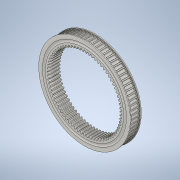
# Autodesk Inventor part: Spur Gear2
Saved by Autodesk Inventor 2020 (Build 240168000, 168)
## iProperties
CustomPartVersion: 1
Created: 2019-05-08
Part Number: Spur Gear2
Material: Steel
Document SubType Name: Modeling
Designer: Connor
Categories: <?xml version="1.0" encoding="UTF-16"?> <MemberInstance><Categories><FamilyTemplate><FamilyTemplateParameter ValueType="xs:double" Id="1" ObjectReferenceKey="da_z" ObjectType="kUserParameterObject"/><FamilyTemplateParameter ValueType="xs:double" Id="2" ObjectReferenceKey="da_b" ObjectType="kUserParameterObject"/><FamilyTemplateParameter ValueType="xs:double" Id="3" ObjectReferenceKey="da_beta" ObjectType="kUserParameterObject"/><FamilyTemplateParameter ValueType="xs:double" Id="4" ObjectReferenceKey="da_da" ObjectType="kUserParameterObject"/><FamilyTemplateParameter ValueType="xs:double" Id="5" ObjectReferenceKey="da_aw" ObjectType="kUserParameterObject"/><FamilyTemplateParameter ValueType="xs:string" Id="6" ObjectReferenceKey="EAIAABAAAAC/AAAAAAAAAIAAAAAAAAAA" ObjectType="83910656" SubObjectId="SurfaceGeometry"/></FamilyTemplate><ParamToTemplateMap><ParamToTemplate CategoryParameter="//CategoryParameter[@InternalName='046C89C9-8512-4d59-83FE-43B91F4F132A']" TemplateParameter="1"/><ParamToTemplate CategoryParameter="//CategoryParameter[@InternalName='2552DF32-E462-4b46-AEBF-C6C7768E72AC']" TemplateParameter="2"/><ParamToTemplate CategoryParameter="//CategoryParameter[@InternalName='C9EE641D-15FC-4fae-A226-E94C4372FDD7']" TemplateParameter="3"/><ParamToTemplate><ParamToTemplate CategoryParameter="//CategoryParameter[@InternalName='00B6519A-459B-49c7-AD84-2E56D39A5744']" ConstantValue="-0.000000"/></ParamToTemplate><ParamToTemplate><ParamToTemplate CategoryParameter="//CategoryParameter[@InternalName='04B31F0E-C7A6-4894-AA32-9629BEFACF47']" ConstantValue="1.000000"/></ParamToTemplate><ParamToTemplate><ParamToTemplate CategoryParameter="//CategoryParameter[@InternalName='43CBEC2E-7847-49e7-A936-2F7889FCB2D9']" ConstantValue="0.250000"/></ParamToTemplate><ParamToTemplate><ParamToTemplate CategoryParameter="//CategoryParameter[@InternalName='B1EFC894-105D-4ebd-86BF-FA20ED196853']" ConstantValue="0.333500"/></ParamToTemplate><ParamToTemplate><ParamToTemplate CategoryParameter="//CategoryParameter[@InternalName='51175063-3D10-4879-93E8-6246FE8B403D']" ConstantValue="2061532430.657340"/></ParamToTemplate><ParamToTemplate><ParamToTemplate CategoryParameter="//CategoryParameter[@InternalName='A3A52E27-4454-46a9-B0BD-C932399B70AF']" ConstantValue="0.300000"/></ParamToTemplate><ParamToTemplate><ParamToTemplate CategoryParameter="//CategoryParameter[@InternalName='91B76062-C214-41d9-B1B9-14D2AB99603D']" ConstantValue="0.127000"/></ParamToTemplate><ParamToTemplate><ParamToTemplate CategoryParameter="//CategoryParameter[@InternalName='374E806E-8B8A-4dda-A9AA-1039D6500AD2']" ConstantValue="7.874016"/></ParamToTemplate><ParamToTemplate><ParamToTemplate CategoryParameter="//CategoryParameter[@InternalName='2D373A89-B862-43d6-8D0B-0CBF12AB9F6C']" ConstantValue="0.253073"/></ParamToTemplate><ParamToTemplate CategoryParameter="//CategoryParameter[@InternalName='37777632-D6A2-4fac-9D53-DB8ACD95C989']" TemplateParameter="4"/><ParamToTemplate CategoryParameter="//CategoryParameter[@InternalName='FD1017F1-B727-4f7e-9707-0F86F1FF9423']" TemplateParameter="5"/><ParamToTemplate><ParamToTemplate CategoryParameter="//CategoryParameter[@InternalName='9E1B4470-B2D3-4ff1-B813-535BB4CDF51A']" ConstantValue="3523220.976809"/></ParamToTemplate><ParamToTemplate><ParamToTemplate CategoryParameter="//CategoryParameter[@InternalName='F8452263-BFF6-458c-9FB1-07C4B99E95CD']" ConstantValue="11397033.805607"/></ParamToTemplate><ParamToTemplate><ParamToTemplate CategoryParameter="//CategoryParameter[@InternalName='3E3BB259-FD49-497f-8171-6EBC954A3479']" ConstantValue="2.000000"/></ParamToTemplate><ParamToTemplate CategoryParameter="//CategoryParameter[@InternalName='27C3BAF2-7550-4e4b-AE2C-0DB134B7D9B7']" TemplateParameter="6"/></ParamToTemplateMap><Category DisplayName="Gear" InternalName="DC85795E-93AB-48d5-8EEE-5A27447B64BD" Mnemonic="Gear"><CategoryParameter DisplayName="z" InternalName="046C89C9-8512-4d59-83FE-43B91F4F132A" Mnemonic="z"/><CategoryParameter DisplayName="b" InternalName="2552DF32-E462-4b46-AEBF-C6C7768E72AC" Mnemonic="b"/><CategoryParameter DisplayName="||b|" InternalName="C9EE641D-15FC-4fae-A226-E94C4372FDD7" Mnemonic="beta"/><CategoryParameter DisplayName="x" InternalName="00B6519A-459B-49c7-AD84-2E56D39A5744" Mnemonic="x"/><CategoryParameter DisplayName="a*" InternalName="04B31F0E-C7A6-4894-AA32-9629BEFACF47" Mnemonic="a"/><CategoryParameter DisplayName="c*" InternalName="43CBEC2E-7847-49e7-A936-2F7889FCB2D9" Mnemonic="c"/><CategoryParameter DisplayName="r|.f|*" InternalName="B1EFC894-105D-4ebd-86BF-FA20ED196853" Mnemonic="rf"/><CategoryParameter DisplayName="E" InternalName="51175063-3D10-4879-93E8-6246FE8B403D" Mnemonic="E"/><CategoryParameter DisplayName="||m|" InternalName="A3A52E27-4454-46a9-B0BD-C932399B70AF" Mnemonic="mi"/><Category DisplayName="SpurGear" InternalName="26C5A22E-A91E-4dfd-A3B3-23CCAFAE1764" Mnemonic="SpurGear"><CategoryParameter DisplayName="m" InternalName="91B76062-C214-41d9-B1B9-14D2AB99603D" Mnemonic="m"/><CategoryParameter DisplayName="P" InternalName="374E806E-8B8A-4dda-A9AA-1039D6500AD2" Mnemonic="PP"/><CategoryParameter DisplayName="||a|" InternalName="2D373A89-B862-43d6-8D0B-0CBF12AB9F6C" Mnemonic="alpha"/><CategoryParameter DisplayName="d|.a|" InternalName="37777632-D6A2-4fac-9D53-DB8ACD95C989" Mnemonic="da"/><CategoryParameter DisplayName="a|.w|" InternalName="FD1017F1-B727-4f7e-9707-0F86F1FF9423" Mnemonic="aw"/><CategoryParameter DisplayName="||s||.Flim|" InternalName="9E1B4470-B2D3-4ff1-B813-535BB4CDF51A" Mnemonic="sFlim"/><CategoryParameter DisplayName="||s||.Hlim|" InternalName="F8452263-BFF6-458c-9FB1-07C4B99E95CD" Mnemonic="sHlim"/><CategoryParameter DisplayName="type" InternalName="3E3BB259-FD49-497f-8171-6EBC954A3479" Mnemonic="type"/><Category DisplayName="InternalSpurGear" InternalName="7CF704F6-14A9-42f8-93CE-E71DF57C2B55" Mnemonic="InternalSpurGear"><CategoryParameter DisplayName="PitchDiameter" InternalName="27C3BAF2-7550-4e4b-AE2C-0DB134B7D9B7" Mnemonic="IDS_PITCHDIAM"/></Category></Category></Category></Categories></MemberInstance>
Density: 1 g/cm^3
Appearance: Steel
Author: Connor
Autodesk Inventor part; units mm, degrees
sketch "Sketch1" plane through (0, 0, 0) normal (0, 0, 1) x (1, 0, 0)
  circle A0 centre (0, 0) radius 52.0383
  dimension "d0" = 104.0765
  constraints: 1 centre point
  measures "d0" diameter of A0
extrude "Extrusion1" add sketch "Sketch1" along normal blind 14
sketch "Sketch2" plane through (0, 0, 0) normal (0, 0, -1) x (-1, 0, 0)
  circle A0 centre (0, 0) radius 52.0383 projected
  circle A1 centre (0, 0) radius 45.72
  dimension "d3" = 91.44
  constraints: 1 centre point, 1 coincident
  measures "d3" diameter of A1
surface extrude "Pitch Diameter" sketch "Sketch2" against normal through all shown no curves A1
ref_plane "Work Plane1" through (0, 0, 0) normal (1, 0, 0) x (0, 1, 0)
ref_plane "Work Plane2" through (0, 0, 0) normal (0.9990482, 0.0436194, 0) x (0, 0, 1)
ref_plane "Work Plane3" through (0, 0, 7) normal (0, 0, -1) x (-1, 0, 0)
spur gear teeth "Spur Gear" teeth 72 pitch diameter 91.44 tip diameter 89.8336 root diameter 94.615 face width 14 start plane through (0, 0, 0) normal (0, 0, -1) x (-1, 0, 0)
sketch "Sketch3" plane through (0, 0, 14) normal (0, 0, 1) x (1, 0, 0)
  circle A0 centre (0, 0) radius 57.3 construction
  circle A1 centre (0, 0) radius 55.22 construction
  line L0 (0, 0) -> (0, 57.3) construction
  circle A2 centre (0, 56.745) radius 1.525 construction
  circle A3 centre (1.9529, 56.8365) radius 0.43 construction
  circle A4 centre (3.0082, 56.7904) radius 0.43 construction
  circle A5 centre (4.9457, 56.5291) radius 1.525 construction
  line L1 (0, 0) -> (4.994, 57.082) construction
  arc A6 (0, 55.22) -> (1.5233, 56.8163) centre (0, 56.745) ccw
  arc A7 (1.9676, 57.2662) -> (1.5233, 56.8163) centre (1.9529, 56.8365) ccw
  arc A8 (3.4343, 56.7329) -> (3.0309, 57.2198) centre (3.0082, 56.7904) ccw
  arc A9 (3.4343, 56.7329) -> (4.8127, 55.0099) centre (4.9457, 56.5291) ccw
  line L2 (1.9676, 57.2662) -> (3.0309, 57.2198)
  arc A10 (-4.8127, 55.0099) -> (-3.4343, 56.7329) centre (-4.9457, 56.5291) ccw
  arc A11 (-3.0309, 57.2198) -> (-3.4343, 56.7329) centre (-3.0082, 56.7904) ccw
  line L3 (-3.0309, 57.2198) -> (-1.9676, 57.2662)
  arc A12 (-1.5233, 56.8163) -> (-1.9676, 57.2662) centre (-1.9529, 56.8365) ccw
  arc A13 (-1.5233, 56.8163) -> (0, 55.22) centre (0, 56.745) ccw
  arc A14 (-9.5889, 54.3811) -> (-8.3659, 56.2177) centre (-9.8537, 55.8829) ccw
  arc A15 (-8.0064, 56.7379) -> (-8.3659, 56.2177) centre (-7.9464, 56.3121) ccw
  line L4 (-8.0064, 56.7379) -> (-6.9512, 56.8768)
  arc A16 (-6.4694, 56.4674) -> (-6.9512, 56.8768) centre (-6.8991, 56.45) ccw
  arc A17 (-6.4694, 56.4674) -> (-4.8127, 55.0099) centre (-4.9457, 56.5291) ccw
  arc A18 (-14.292, 53.3384) -> (-13.2337, 55.2746) centre (-14.6867, 54.8115) ccw
  arc A19 (-12.921, 55.8242) -> (-13.2337, 55.2746) centre (-12.824, 55.4052) ccw
  line L5 (-12.921, 55.8242) -> (-11.8819, 56.0545)
  arc A20 (-11.3662, 55.6887) -> (-11.8819, 56.0545) centre (-11.7927, 55.6339) ccw
  arc A21 (-11.3662, 55.6887) -> (-9.5889, 54.3811) centre (-9.8537, 55.8829) ccw
  arc A22 (-18.8864, 51.8898) -> (-18.0009, 53.9109) centre (-19.4079, 53.3229) ccw
  arc A23 (-17.7372, 54.4856) -> (-18.0009, 53.9109) centre (-17.6041, 54.0767) ccw
  line L6 (-17.7372, 54.4856) -> (-16.7222, 54.8056)
  arc A24 (-16.1766, 54.4861) -> (-16.7222, 54.8056) centre (-16.5967, 54.3944) ccw
  arc A25 (-16.1766, 54.4861) -> (-14.292, 53.3384) centre (-14.6867, 54.8115) ccw
  arc A26 (-23.337, 50.0463) -> (-22.631, 52.1369) centre (-23.9815, 51.4284) ccw
  arc A27 (-22.4185, 52.7324) -> (-22.631, 52.1369) centre (-22.2502, 52.3366) ccw
  line L7 (-22.4185, 52.7324) -> (-21.4352, 53.1397)
  arc A28 (-20.8638, 52.8689) -> (-21.4352, 53.1397) centre (-21.2743, 52.7409) ccw
  arc A29 (-20.8638, 52.8689) -> (-18.8864, 51.8898) centre (-19.4079, 53.3229) ccw
  arc A30 (-27.61, 47.8219) -> (-27.0889, 49.9661) centre (-28.3725, 49.1426) ccw
  arc A31 (-26.9291, 50.5778) -> (-27.0889, 49.9661) centre (-26.727, 50.1982) ccw
  line L8 (-26.9291, 50.5778) -> (-25.985, 51.0693)
  arc A32 (-25.3922, 50.8493) -> (-25.985, 51.0693) centre (-25.79, 50.686) ccw
  arc A33 (-25.3922, 50.8493) -> (-23.337, 50.0463) centre (-23.9815, 51.4284) ccw
  arc A34 (-31.6729, 45.2336) -> (-31.3407, 47.415) centre (-32.5476, 46.4828) ccw
  arc A35 (-31.2348, 48.0383) -> (-31.3407, 47.415) centre (-31.0004, 47.6778) ccw
  line L9 (-31.2348, 48.0383) -> (-30.3371, 48.6102)
  arc A36 (-29.7274, 48.4427) -> (-30.3371, 48.6102) centre (-30.1095, 48.2454) ccw
  arc A37 (-29.7274, 48.4427) -> (-27.61, 47.8219) centre (-28.3725, 49.1426) ccw
  arc A38 (-35.4947, 42.301) -> (-35.3539, 44.503) centre (-36.475, 43.4692) ccw
  arc A39 (-35.3027, 45.1332) -> (-35.3539, 44.503) centre (-35.0378, 44.7945) ccw
  line L10 (-35.3027, 45.1332) -> (-34.4583, 45.7811)
  arc A40 (-33.8364, 45.6675) -> (-34.4583, 45.7811) centre (-34.1997, 45.4376) ccw
  arc A41 (-33.8364, 45.6675) -> (-31.6729, 45.2336) centre (-32.5476, 46.4828) ccw
  arc A42 (-39.0464, 39.0464) -> (-39.0981, 41.2524) centre (-40.1248, 40.1248) ccw
  arc A43 (-39.102, 41.8846) -> (-39.0981, 41.2524) centre (-38.8086, 41.5703) ccw
  line L11 (-39.102, 41.8846) -> (-38.3173, 42.6037)
  arc A44 (-37.6878, 42.5447) -> (-38.3173, 42.6037) centre (-38.0297, 42.284) ccw
  arc A45 (-37.6878, 42.5447) -> (-35.4947, 42.301) centre (-36.475, 43.4692) ccw
  arc A46 (-42.301, 35.4947) -> (-42.5447, 37.6878) centre (-43.4692, 36.475) ccw
  arc A47 (-42.6037, 38.3173) -> (-42.5447, 37.6878) centre (-42.284, 38.0297) ccw
  line L12 (-42.6037, 38.3173) -> (-41.8846, 39.102)
  arc A48 (-41.2524, 39.0981) -> (-41.8846, 39.102) centre (-41.5703, 38.8086) ccw
  arc A49 (-41.2524, 39.0981) -> (-39.0464, 39.0464) centre (-40.1248, 40.1248) ccw
  arc A50 (-45.2336, 31.6729) -> (-45.6675, 33.8364) centre (-46.4828, 32.5476) ccw
  arc A51 (-45.7811, 34.4583) -> (-45.6675, 33.8364) centre (-45.4376, 34.1997) ccw
  line L13 (-45.7811, 34.4583) -> (-45.1332, 35.3027)
  arc A52 (-44.503, 35.3539) -> (-45.1332, 35.3027) centre (-44.7945, 35.0378) ccw
  arc A53 (-44.503, 35.3539) -> (-42.301, 35.4947) centre (-43.4692, 36.475) ccw
  arc A54 (-47.8219, 27.61) -> (-48.4427, 29.7274) centre (-49.1426, 28.3725) ccw
  arc A55 (-48.6102, 30.3371) -> (-48.4427, 29.7274) centre (-48.2454, 30.1095) ccw
  line L14 (-48.6102, 30.3371) -> (-48.0383, 31.2348)
  arc A56 (-47.415, 31.3407) -> (-48.0383, 31.2348) centre (-47.6778, 31.0004) ccw
  arc A57 (-47.415, 31.3407) -> (-45.2336, 31.6729) centre (-46.4828, 32.5476) ccw
  arc A58 (-50.0463, 23.337) -> (-50.8493, 25.3922) centre (-51.4284, 23.9815) ccw
  arc A59 (-51.0693, 25.985) -> (-50.8493, 25.3922) centre (-50.686, 25.79) ccw
  line L15 (-51.0693, 25.985) -> (-50.5778, 26.9291)
  arc A60 (-49.9661, 27.0889) -> (-50.5778, 26.9291) centre (-50.1982, 26.727) ccw
  arc A61 (-49.9661, 27.0889) -> (-47.8219, 27.61) centre (-49.1426, 28.3725) ccw
  arc A62 (-51.8898, 18.8864) -> (-52.8689, 20.8638) centre (-53.3229, 19.4079) ccw
  arc A63 (-53.1397, 21.4352) -> (-52.8689, 20.8638) centre (-52.7409, 21.2743) ccw
  line L16 (-53.1397, 21.4352) -> (-52.7324, 22.4185)
  arc A64 (-52.1369, 22.631) -> (-52.7324, 22.4185) centre (-52.3366, 22.2502) ccw
  arc A65 (-52.1369, 22.631) -> (-50.0463, 23.337) centre (-51.4284, 23.9815) ccw
  arc A66 (-53.3384, 14.292) -> (-54.4861, 16.1766) centre (-54.8115, 14.6867) ccw
  arc A67 (-54.8056, 16.7222) -> (-54.4861, 16.1766) centre (-54.3944, 16.5967) ccw
  line L17 (-54.8056, 16.7222) -> (-54.4856, 17.7372)
  arc A68 (-53.9109, 18.0009) -> (-54.4856, 17.7372) centre (-54.0767, 17.6041) ccw
  arc A69 (-53.9109, 18.0009) -> (-51.8898, 18.8864) centre (-53.3229, 19.4079) ccw
  arc A70 (-54.3811, 9.5889) -> (-55.6887, 11.3662) centre (-55.8829, 9.8537) ccw
  arc A71 (-56.0545, 11.8819) -> (-55.6887, 11.3662) centre (-55.6339, 11.7927) ccw
  line L18 (-56.0545, 11.8819) -> (-55.8242, 12.921)
  arc A72 (-55.2746, 13.2337) -> (-55.8242, 12.921) centre (-55.4052, 12.824) ccw
  arc A73 (-55.2746, 13.2337) -> (-53.3384, 14.292) centre (-54.8115, 14.6867) ccw
  arc A74 (-55.0099, 4.8127) -> (-56.4674, 6.4694) centre (-56.5291, 4.9457) ccw
  arc A75 (-56.8768, 6.9512) -> (-56.4674, 6.4694) centre (-56.45, 6.8991) ccw
  line L19 (-56.8768, 6.9512) -> (-56.7379, 8.0064)
  arc A76 (-56.2177, 8.3659) -> (-56.7379, 8.0064) centre (-56.3121, 7.9464) ccw
  arc A77 (-56.2177, 8.3659) -> (-54.3811, 9.5889) centre (-55.8829, 9.8537) ccw
  arc A78 (-55.22, 0) -> (-56.8163, 1.5233) centre (-56.745, 0) ccw
  arc A79 (-57.2662, 1.9676) -> (-56.8163, 1.5233) centre (-56.8365, 1.9529) ccw
  line L20 (-57.2662, 1.9676) -> (-57.2198, 3.0309)
  arc A80 (-56.7329, 3.4343) -> (-57.2198, 3.0309) centre (-56.7904, 3.0082) ccw
  arc A81 (-56.7329, 3.4343) -> (-55.0099, 4.8127) centre (-56.5291, 4.9457) ccw
  arc A82 (-55.0099, -4.8127) -> (-56.7329, -3.4343) centre (-56.5291, -4.9457) ccw
  arc A83 (-57.2198, -3.0309) -> (-56.7329, -3.4343) centre (-56.7904, -3.0082) ccw
  line L21 (-57.2198, -3.0309) -> (-57.2662, -1.9676)
  arc A84 (-56.8163, -1.5233) -> (-57.2662, -1.9676) centre (-56.8365, -1.9529) ccw
  arc A85 (-56.8163, -1.5233) -> (-55.22, 0) centre (-56.745, 0) ccw
  arc A86 (-54.3811, -9.5889) -> (-56.2177, -8.3659) centre (-55.8829, -9.8537) ccw
  arc A87 (-56.7379, -8.0064) -> (-56.2177, -8.3659) centre (-56.3121, -7.9464) ccw
  line L22 (-56.7379, -8.0064) -> (-56.8768, -6.9512)
  arc A88 (-56.4674, -6.4694) -> (-56.8768, -6.9512) centre (-56.45, -6.8991) ccw
  arc A89 (-56.4674, -6.4694) -> (-55.0099, -4.8127) centre (-56.5291, -4.9457) ccw
  arc A90 (-53.3384, -14.292) -> (-55.2746, -13.2337) centre (-54.8115, -14.6867) ccw
  arc A91 (-55.8242, -12.921) -> (-55.2746, -13.2337) centre (-55.4052, -12.824) ccw
  line L23 (-55.8242, -12.921) -> (-56.0545, -11.8819)
  arc A92 (-55.6887, -11.3662) -> (-56.0545, -11.8819) centre (-55.6339, -11.7927) ccw
  arc A93 (-55.6887, -11.3662) -> (-54.3811, -9.5889) centre (-55.8829, -9.8537) ccw
  arc A94 (-51.8898, -18.8864) -> (-53.9109, -18.0009) centre (-53.3229, -19.4079) ccw
  arc A95 (-54.4856, -17.7372) -> (-53.9109, -18.0009) centre (-54.0767, -17.6041) ccw
  line L24 (-54.4856, -17.7372) -> (-54.8056, -16.7222)
  arc A96 (-54.4861, -16.1766) -> (-54.8056, -16.7222) centre (-54.3944, -16.5967) ccw
  arc A97 (-54.4861, -16.1766) -> (-53.3384, -14.292) centre (-54.8115, -14.6867) ccw
  arc A98 (-50.0463, -23.337) -> (-52.1369, -22.631) centre (-51.4284, -23.9815) ccw
  arc A99 (-52.7324, -22.4185) -> (-52.1369, -22.631) centre (-52.3366, -22.2502) ccw
  line L25 (-52.7324, -22.4185) -> (-53.1397, -21.4352)
  arc A100 (-52.8689, -20.8638) -> (-53.1397, -21.4352) centre (-52.7409, -21.2743) ccw
  arc A101 (-52.8689, -20.8638) -> (-51.8898, -18.8864) centre (-53.3229, -19.4079) ccw
  arc A102 (-47.8219, -27.61) -> (-49.9661, -27.0889) centre (-49.1426, -28.3725) ccw
  arc A103 (-50.5778, -26.9291) -> (-49.9661, -27.0889) centre (-50.1982, -26.727) ccw
  line L26 (-50.5778, -26.9291) -> (-51.0693, -25.985)
  arc A104 (-50.8493, -25.3922) -> (-51.0693, -25.985) centre (-50.686, -25.79) ccw
  arc A105 (-50.8493, -25.3922) -> (-50.0463, -23.337) centre (-51.4284, -23.9815) ccw
  arc A106 (-45.2336, -31.6729) -> (-47.415, -31.3407) centre (-46.4828, -32.5476) ccw
  arc A107 (-48.0383, -31.2348) -> (-47.415, -31.3407) centre (-47.6778, -31.0004) ccw
  line L27 (-48.0383, -31.2348) -> (-48.6102, -30.3371)
  arc A108 (-48.4427, -29.7274) -> (-48.6102, -30.3371) centre (-48.2454, -30.1095) ccw
  arc A109 (-48.4427, -29.7274) -> (-47.8219, -27.61) centre (-49.1426, -28.3725) ccw
  arc A110 (-42.301, -35.4947) -> (-44.503, -35.3539) centre (-43.4692, -36.475) ccw
  arc A111 (-45.1332, -35.3027) -> (-44.503, -35.3539) centre (-44.7945, -35.0378) ccw
  line L28 (-45.1332, -35.3027) -> (-45.7811, -34.4583)
  arc A112 (-45.6675, -33.8364) -> (-45.7811, -34.4583) centre (-45.4376, -34.1997) ccw
  arc A113 (-45.6675, -33.8364) -> (-45.2336, -31.6729) centre (-46.4828, -32.5476) ccw
  arc A114 (-39.0464, -39.0464) -> (-41.2524, -39.0981) centre (-40.1248, -40.1248) ccw
  arc A115 (-41.8846, -39.102) -> (-41.2524, -39.0981) centre (-41.5703, -38.8086) ccw
  line L29 (-41.8846, -39.102) -> (-42.6037, -38.3173)
  arc A116 (-42.5447, -37.6878) -> (-42.6037, -38.3173) centre (-42.284, -38.0297) ccw
  arc A117 (-42.5447, -37.6878) -> (-42.301, -35.4947) centre (-43.4692, -36.475) ccw
  arc A118 (-35.4947, -42.301) -> (-37.6878, -42.5447) centre (-36.475, -43.4692) ccw
  arc A119 (-38.3173, -42.6037) -> (-37.6878, -42.5447) centre (-38.0297, -42.284) ccw
  line L30 (-38.3173, -42.6037) -> (-39.102, -41.8846)
  arc A120 (-39.0981, -41.2524) -> (-39.102, -41.8846) centre (-38.8086, -41.5703) ccw
  arc A121 (-39.0981, -41.2524) -> (-39.0464, -39.0464) centre (-40.1248, -40.1248) ccw
  arc A122 (-31.6729, -45.2336) -> (-33.8364, -45.6675) centre (-32.5476, -46.4828) ccw
  arc A123 (-34.4583, -45.7811) -> (-33.8364, -45.6675) centre (-34.1997, -45.4376) ccw
  line L31 (-34.4583, -45.7811) -> (-35.3027, -45.1332)
  arc A124 (-35.3539, -44.503) -> (-35.3027, -45.1332) centre (-35.0378, -44.7945) ccw
  arc A125 (-35.3539, -44.503) -> (-35.4947, -42.301) centre (-36.475, -43.4692) ccw
  arc A126 (-27.61, -47.8219) -> (-29.7274, -48.4427) centre (-28.3725, -49.1426) ccw
  arc A127 (-30.3371, -48.6102) -> (-29.7274, -48.4427) centre (-30.1095, -48.2454) ccw
  line L32 (-30.3371, -48.6102) -> (-31.2348, -48.0383)
  arc A128 (-31.3407, -47.415) -> (-31.2348, -48.0383) centre (-31.0004, -47.6778) ccw
  arc A129 (-31.3407, -47.415) -> (-31.6729, -45.2336) centre (-32.5476, -46.4828) ccw
  arc A130 (-23.337, -50.0463) -> (-25.3922, -50.8493) centre (-23.9815, -51.4284) ccw
  arc A131 (-25.985, -51.0693) -> (-25.3922, -50.8493) centre (-25.79, -50.686) ccw
  line L33 (-25.985, -51.0693) -> (-26.9291, -50.5778)
  arc A132 (-27.0889, -49.9661) -> (-26.9291, -50.5778) centre (-26.727, -50.1982) ccw
  arc A133 (-27.0889, -49.9661) -> (-27.61, -47.8219) centre (-28.3725, -49.1426) ccw
  arc A134 (-18.8864, -51.8898) -> (-20.8638, -52.8689) centre (-19.4079, -53.3229) ccw
  arc A135 (-21.4352, -53.1397) -> (-20.8638, -52.8689) centre (-21.2743, -52.7409) ccw
  line L34 (-21.4352, -53.1397) -> (-22.4185, -52.7324)
  arc A136 (-22.631, -52.1369) -> (-22.4185, -52.7324) centre (-22.2502, -52.3366) ccw
  arc A137 (-22.631, -52.1369) -> (-23.337, -50.0463) centre (-23.9815, -51.4284) ccw
  arc A138 (-14.292, -53.3384) -> (-16.1766, -54.4861) centre (-14.6867, -54.8115) ccw
  arc A139 (-16.7222, -54.8056) -> (-16.1766, -54.4861) centre (-16.5967, -54.3944) ccw
  line L35 (-16.7222, -54.8056) -> (-17.7372, -54.4856)
  arc A140 (-18.0009, -53.9109) -> (-17.7372, -54.4856) centre (-17.6041, -54.0767) ccw
  arc A141 (-18.0009, -53.9109) -> (-18.8864, -51.8898) centre (-19.4079, -53.3229) ccw
  arc A142 (-9.5889, -54.3811) -> (-11.3662, -55.6887) centre (-9.8537, -55.8829) ccw
  arc A143 (-11.8819, -56.0545) -> (-11.3662, -55.6887) centre (-11.7927, -55.6339) ccw
  line L36 (-11.8819, -56.0545) -> (-12.921, -55.8242)
  arc A144 (-13.2337, -55.2746) -> (-12.921, -55.8242) centre (-12.824, -55.4052) ccw
  arc A145 (-13.2337, -55.2746) -> (-14.292, -53.3384) centre (-14.6867, -54.8115) ccw
  arc A146 (-4.8127, -55.0099) -> (-6.4694, -56.4674) centre (-4.9457, -56.5291) ccw
  arc A147 (-6.9512, -56.8768) -> (-6.4694, -56.4674) centre (-6.8991, -56.45) ccw
  line L37 (-6.9512, -56.8768) -> (-8.0064, -56.7379)
  arc A148 (-8.3659, -56.2177) -> (-8.0064, -56.7379) centre (-7.9464, -56.3121) ccw
  arc A149 (-8.3659, -56.2177) -> (-9.5889, -54.3811) centre (-9.8537, -55.8829) ccw
  arc A150 (0, -55.22) -> (-1.5233, -56.8163) centre (0, -56.745) ccw
  arc A151 (-1.9676, -57.2662) -> (-1.5233, -56.8163) centre (-1.9529, -56.8365) ccw
  line L38 (-1.9676, -57.2662) -> (-3.0309, -57.2198)
  arc A152 (-3.4343, -56.7329) -> (-3.0309, -57.2198) centre (-3.0082, -56.7904) ccw
  arc A153 (-3.4343, -56.7329) -> (-4.8127, -55.0099) centre (-4.9457, -56.5291) ccw
  arc A154 (4.8127, -55.0099) -> (3.4343, -56.7329) centre (4.9457, -56.5291) ccw
  arc A155 (3.0309, -57.2198) -> (3.4343, -56.7329) centre (3.0082, -56.7904) ccw
  line L39 (3.0309, -57.2198) -> (1.9676, -57.2662)
  arc A156 (1.5233, -56.8163) -> (1.9676, -57.2662) centre (1.9529, -56.8365) ccw
  arc A157 (1.5233, -56.8163) -> (0, -55.22) centre (0, -56.745) ccw
  arc A158 (9.5889, -54.3811) -> (8.3659, -56.2177) centre (9.8537, -55.8829) ccw
  arc A159 (8.0064, -56.7379) -> (8.3659, -56.2177) centre (7.9464, -56.3121) ccw
  line L40 (8.0064, -56.7379) -> (6.9512, -56.8768)
  arc A160 (6.4694, -56.4674) -> (6.9512, -56.8768) centre (6.8991, -56.45) ccw
  arc A161 (6.4694, -56.4674) -> (4.8127, -55.0099) centre (4.9457, -56.5291) ccw
  arc A162 (14.292, -53.3384) -> (13.2337, -55.2746) centre (14.6867, -54.8115) ccw
  arc A163 (12.921, -55.8242) -> (13.2337, -55.2746) centre (12.824, -55.4052) ccw
  line L41 (12.921, -55.8242) -> (11.8819, -56.0545)
  arc A164 (11.3662, -55.6887) -> (11.8819, -56.0545) centre (11.7927, -55.6339) ccw
  arc A165 (11.3662, -55.6887) -> (9.5889, -54.3811) centre (9.8537, -55.8829) ccw
  arc A166 (18.8864, -51.8898) -> (18.0009, -53.9109) centre (19.4079, -53.3229) ccw
  arc A167 (17.7372, -54.4856) -> (18.0009, -53.9109) centre (17.6041, -54.0767) ccw
  line L42 (17.7372, -54.4856) -> (16.7222, -54.8056)
  arc A168 (16.1766, -54.4861) -> (16.7222, -54.8056) centre (16.5967, -54.3944) ccw
  arc A169 (16.1766, -54.4861) -> (14.292, -53.3384) centre (14.6867, -54.8115) ccw
  arc A170 (23.337, -50.0463) -> (22.631, -52.1369) centre (23.9815, -51.4284) ccw
  arc A171 (22.4185, -52.7324) -> (22.631, -52.1369) centre (22.2502, -52.3366) ccw
  line L43 (22.4185, -52.7324) -> (21.4352, -53.1397)
  arc A172 (20.8638, -52.8689) -> (21.4352, -53.1397) centre (21.2743, -52.7409) ccw
  arc A173 (20.8638, -52.8689) -> (18.8864, -51.8898) centre (19.4079, -53.3229) ccw
  arc A174 (27.61, -47.8219) -> (27.0889, -49.9661) centre (28.3725, -49.1426) ccw
  arc A175 (26.9291, -50.5778) -> (27.0889, -49.9661) centre (26.727, -50.1982) ccw
  line L44 (26.9291, -50.5778) -> (25.985, -51.0693)
  arc A176 (25.3922, -50.8493) -> (25.985, -51.0693) centre (25.79, -50.686) ccw
  arc A177 (25.3922, -50.8493) -> (23.337, -50.0463) centre (23.9815, -51.4284) ccw
  arc A178 (31.6729, -45.2336) -> (31.3407, -47.415) centre (32.5476, -46.4828) ccw
  arc A179 (31.2348, -48.0383) -> (31.3407, -47.415) centre (31.0004, -47.6778) ccw
  line L45 (31.2348, -48.0383) -> (30.3371, -48.6102)
  arc A180 (29.7274, -48.4427) -> (30.3371, -48.6102) centre (30.1095, -48.2454) ccw
  arc A181 (29.7274, -48.4427) -> (27.61, -47.8219) centre (28.3725, -49.1426) ccw
  arc A182 (35.4947, -42.301) -> (35.3539, -44.503) centre (36.475, -43.4692) ccw
  arc A183 (35.3027, -45.1332) -> (35.3539, -44.503) centre (35.0378, -44.7945) ccw
  line L46 (35.3027, -45.1332) -> (34.4583, -45.7811)
  arc A184 (33.8364, -45.6675) -> (34.4583, -45.7811) centre (34.1997, -45.4376) ccw
  arc A185 (33.8364, -45.6675) -> (31.6729, -45.2336) centre (32.5476, -46.4828) ccw
  arc A186 (39.0464, -39.0464) -> (39.0981, -41.2524) centre (40.1248, -40.1248) ccw
  arc A187 (39.102, -41.8846) -> (39.0981, -41.2524) centre (38.8086, -41.5703) ccw
  line L47 (39.102, -41.8846) -> (38.3173, -42.6037)
  arc A188 (37.6878, -42.5447) -> (38.3173, -42.6037) centre (38.0297, -42.284) ccw
  arc A189 (37.6878, -42.5447) -> (35.4947, -42.301) centre (36.475, -43.4692) ccw
  arc A190 (42.301, -35.4947) -> (42.5447, -37.6878) centre (43.4692, -36.475) ccw
  arc A191 (42.6037, -38.3173) -> (42.5447, -37.6878) centre (42.284, -38.0297) ccw
  line L48 (42.6037, -38.3173) -> (41.8846, -39.102)
  arc A192 (41.2524, -39.0981) -> (41.8846, -39.102) centre (41.5703, -38.8086) ccw
  arc A193 (41.2524, -39.0981) -> (39.0464, -39.0464) centre (40.1248, -40.1248) ccw
  arc A194 (45.2336, -31.6729) -> (45.6675, -33.8364) centre (46.4828, -32.5476) ccw
  arc A195 (45.7811, -34.4583) -> (45.6675, -33.8364) centre (45.4376, -34.1997) ccw
  line L49 (45.7811, -34.4583) -> (45.1332, -35.3027)
  arc A196 (44.503, -35.3539) -> (45.1332, -35.3027) centre (44.7945, -35.0378) ccw
  arc A197 (44.503, -35.3539) -> (42.301, -35.4947) centre (43.4692, -36.475) ccw
  arc A198 (47.8219, -27.61) -> (48.4427, -29.7274) centre (49.1426, -28.3725) ccw
  arc A199 (48.6102, -30.3371) -> (48.4427, -29.7274) centre (48.2454, -30.1095) ccw
  line L50 (48.6102, -30.3371) -> (48.0383, -31.2348)
  arc A200 (47.415, -31.3407) -> (48.0383, -31.2348) centre (47.6778, -31.0004) ccw
  arc A201 (47.415, -31.3407) -> (45.2336, -31.6729) centre (46.4828, -32.5476) ccw
  arc A202 (50.0463, -23.337) -> (50.8493, -25.3922) centre (51.4284, -23.9815) ccw
  arc A203 (51.0693, -25.985) -> (50.8493, -25.3922) centre (50.686, -25.79) ccw
  line L51 (51.0693, -25.985) -> (50.5778, -26.9291)
  arc A204 (49.9661, -27.0889) -> (50.5778, -26.9291) centre (50.1982, -26.727) ccw
  arc A205 (49.9661, -27.0889) -> (47.8219, -27.61) centre (49.1426, -28.3725) ccw
  arc A206 (51.8898, -18.8864) -> (52.8689, -20.8638) centre (53.3229, -19.4079) ccw
  arc A207 (53.1397, -21.4352) -> (52.8689, -20.8638) centre (52.7409, -21.2743) ccw
  line L52 (53.1397, -21.4352) -> (52.7324, -22.4185)
  arc A208 (52.1369, -22.631) -> (52.7324, -22.4185) centre (52.3366, -22.2502) ccw
  arc A209 (52.1369, -22.631) -> (50.0463, -23.337) centre (51.4284, -23.9815) ccw
  arc A210 (53.3384, -14.292) -> (54.4861, -16.1766) centre (54.8115, -14.6867) ccw
  arc A211 (54.8056, -16.7222) -> (54.4861, -16.1766) centre (54.3944, -16.5967) ccw
  line L53 (54.8056, -16.7222) -> (54.4856, -17.7372)
  arc A212 (53.9109, -18.0009) -> (54.4856, -17.7372) centre (54.0767, -17.6041) ccw
  arc A213 (53.9109, -18.0009) -> (51.8898, -18.8864) centre (53.3229, -19.4079) ccw
  arc A214 (54.3811, -9.5889) -> (55.6887, -11.3662) centre (55.8829, -9.8537) ccw
  arc A215 (56.0545, -11.8819) -> (55.6887, -11.3662) centre (55.6339, -11.7927) ccw
  line L54 (56.0545, -11.8819) -> (55.8242, -12.921)
  arc A216 (55.2746, -13.2337) -> (55.8242, -12.921) centre (55.4052, -12.824) ccw
  arc A217 (55.2746, -13.2337) -> (53.3384, -14.292) centre (54.8115, -14.6867) ccw
  arc A218 (55.0099, -4.8127) -> (56.4674, -6.4694) centre (56.5291, -4.9457) ccw
  arc A219 (56.8768, -6.9512) -> (56.4674, -6.4694) centre (56.45, -6.8991) ccw
  line L55 (56.8768, -6.9512) -> (56.7379, -8.0064)
  arc A220 (56.2177, -8.3659) -> (56.7379, -8.0064) centre (56.3121, -7.9464) ccw
  arc A221 (56.2177, -8.3659) -> (54.3811, -9.5889) centre (55.8829, -9.8537) ccw
  arc A222 (55.22, 0) -> (56.8163, -1.5233) centre (56.745, 0) ccw
  arc A223 (57.2662, -1.9676) -> (56.8163, -1.5233) centre (56.8365, -1.9529) ccw
  line L56 (57.2662, -1.9676) -> (57.2198, -3.0309)
  arc A224 (56.7329, -3.4343) -> (57.2198, -3.0309) centre (56.7904, -3.0082) ccw
  arc A225 (56.7329, -3.4343) -> (55.0099, -4.8127) centre (56.5291, -4.9457) ccw
  arc A226 (55.0099, 4.8127) -> (56.7329, 3.4343) centre (56.5291, 4.9457) ccw
  arc A227 (57.2198, 3.0309) -> (56.7329, 3.4343) centre (56.7904, 3.0082) ccw
  line L57 (57.2198, 3.0309) -> (57.2662, 1.9676)
  arc A228 (56.8163, 1.5233) -> (57.2662, 1.9676) centre (56.8365, 1.9529) ccw
  arc A229 (56.8163, 1.5233) -> (55.22, 0) centre (56.745, 0) ccw
  arc A230 (54.3811, 9.5889) -> (56.2177, 8.3659) centre (55.8829, 9.8537) ccw
  arc A231 (56.7379, 8.0064) -> (56.2177, 8.3659) centre (56.3121, 7.9464) ccw
  line L58 (56.7379, 8.0064) -> (56.8768, 6.9512)
  arc A232 (56.4674, 6.4694) -> (56.8768, 6.9512) centre (56.45, 6.8991) ccw
  arc A233 (56.4674, 6.4694) -> (55.0099, 4.8127) centre (56.5291, 4.9457) ccw
  arc A234 (53.3384, 14.292) -> (55.2746, 13.2337) centre (54.8115, 14.6867) ccw
  arc A235 (55.8242, 12.921) -> (55.2746, 13.2337) centre (55.4052, 12.824) ccw
  line L59 (55.8242, 12.921) -> (56.0545, 11.8819)
  arc A236 (55.6887, 11.3662) -> (56.0545, 11.8819) centre (55.6339, 11.7927) ccw
  arc A237 (55.6887, 11.3662) -> (54.3811, 9.5889) centre (55.8829, 9.8537) ccw
  arc A238 (51.8898, 18.8864) -> (53.9109, 18.0009) centre (53.3229, 19.4079) ccw
  arc A239 (54.4856, 17.7372) -> (53.9109, 18.0009) centre (54.0767, 17.6041) ccw
  line L60 (54.4856, 17.7372) -> (54.8056, 16.7222)
  arc A240 (54.4861, 16.1766) -> (54.8056, 16.7222) centre (54.3944, 16.5967) ccw
  arc A241 (54.4861, 16.1766) -> (53.3384, 14.292) centre (54.8115, 14.6867) ccw
  arc A242 (50.0463, 23.337) -> (52.1369, 22.631) centre (51.4284, 23.9815) ccw
  arc A243 (52.7324, 22.4185) -> (52.1369, 22.631) centre (52.3366, 22.2502) ccw
  line L61 (52.7324, 22.4185) -> (53.1397, 21.4352)
  arc A244 (52.8689, 20.8638) -> (53.1397, 21.4352) centre (52.7409, 21.2743) ccw
  arc A245 (52.8689, 20.8638) -> (51.8898, 18.8864) centre (53.3229, 19.4079) ccw
  arc A246 (47.8219, 27.61) -> (49.9661, 27.0889) centre (49.1426, 28.3725) ccw
  arc A247 (50.5778, 26.9291) -> (49.9661, 27.0889) centre (50.1982, 26.727) ccw
  line L62 (50.5778, 26.9291) -> (51.0693, 25.985)
  arc A248 (50.8493, 25.3922) -> (51.0693, 25.985) centre (50.686, 25.79) ccw
  arc A249 (50.8493, 25.3922) -> (50.0463, 23.337) centre (51.4284, 23.9815) ccw
  arc A250 (45.2336, 31.6729) -> (47.415, 31.3407) centre (46.4828, 32.5476) ccw
  arc A251 (48.0383, 31.2348) -> (47.415, 31.3407) centre (47.6778, 31.0004) ccw
  line L63 (48.0383, 31.2348) -> (48.6102, 30.3371)
  arc A252 (48.4427, 29.7274) -> (48.6102, 30.3371) centre (48.2454, 30.1095) ccw
  arc A253 (48.4427, 29.7274) -> (47.8219, 27.61) centre (49.1426, 28.3725) ccw
  arc A254 (42.301, 35.4947) -> (44.503, 35.3539) centre (43.4692, 36.475) ccw
  arc A255 (45.1332, 35.3027) -> (44.503, 35.3539) centre (44.7945, 35.0378) ccw
  line L64 (45.1332, 35.3027) -> (45.7811, 34.4583)
  arc A256 (45.6675, 33.8364) -> (45.7811, 34.4583) centre (45.4376, 34.1997) ccw
  arc A257 (45.6675, 33.8364) -> (45.2336, 31.6729) centre (46.4828, 32.5476) ccw
  arc A258 (39.0464, 39.0464) -> (41.2524, 39.0981) centre (40.1248, 40.1248) ccw
  arc A259 (41.8846, 39.102) -> (41.2524, 39.0981) centre (41.5703, 38.8086) ccw
  line L65 (41.8846, 39.102) -> (42.6037, 38.3173)
  arc A260 (42.5447, 37.6878) -> (42.6037, 38.3173) centre (42.284, 38.0297) ccw
  arc A261 (42.5447, 37.6878) -> (42.301, 35.4947) centre (43.4692, 36.475) ccw
  arc A262 (35.4947, 42.301) -> (37.6878, 42.5447) centre (36.475, 43.4692) ccw
  arc A263 (38.3173, 42.6037) -> (37.6878, 42.5447) centre (38.0297, 42.284) ccw
  line L66 (38.3173, 42.6037) -> (39.102, 41.8846)
  arc A264 (39.0981, 41.2524) -> (39.102, 41.8846) centre (38.8086, 41.5703) ccw
  arc A265 (39.0981, 41.2524) -> (39.0464, 39.0464) centre (40.1248, 40.1248) ccw
  arc A266 (31.6729, 45.2336) -> (33.8364, 45.6675) centre (32.5476, 46.4828) ccw
  arc A267 (34.4583, 45.7811) -> (33.8364, 45.6675) centre (34.1997, 45.4376) ccw
  line L67 (34.4583, 45.7811) -> (35.3027, 45.1332)
  arc A268 (35.3539, 44.503) -> (35.3027, 45.1332) centre (35.0378, 44.7945) ccw
  arc A269 (35.3539, 44.503) -> (35.4947, 42.301) centre (36.475, 43.4692) ccw
  arc A270 (27.61, 47.8219) -> (29.7274, 48.4427) centre (28.3725, 49.1426) ccw
  arc A271 (30.3371, 48.6102) -> (29.7274, 48.4427) centre (30.1095, 48.2454) ccw
  line L68 (30.3371, 48.6102) -> (31.2348, 48.0383)
  arc A272 (31.3407, 47.415) -> (31.2348, 48.0383) centre (31.0004, 47.6778) ccw
  arc A273 (31.3407, 47.415) -> (31.6729, 45.2336) centre (32.5476, 46.4828) ccw
  arc A274 (23.337, 50.0463) -> (25.3922, 50.8493) centre (23.9815, 51.4284) ccw
  arc A275 (25.985, 51.0693) -> (25.3922, 50.8493) centre (25.79, 50.686) ccw
  line L69 (25.985, 51.0693) -> (26.9291, 50.5778)
  arc A276 (27.0889, 49.9661) -> (26.9291, 50.5778) centre (26.727, 50.1982) ccw
  arc A277 (27.0889, 49.9661) -> (27.61, 47.8219) centre (28.3725, 49.1426) ccw
  arc A278 (18.8864, 51.8898) -> (20.8638, 52.8689) centre (19.4079, 53.3229) ccw
  arc A279 (21.4352, 53.1397) -> (20.8638, 52.8689) centre (21.2743, 52.7409) ccw
  line L70 (21.4352, 53.1397) -> (22.4185, 52.7324)
  arc A280 (22.631, 52.1369) -> (22.4185, 52.7324) centre (22.2502, 52.3366) ccw
  arc A281 (22.631, 52.1369) -> (23.337, 50.0463) centre (23.9815, 51.4284) ccw
  arc A282 (14.292, 53.3384) -> (16.1766, 54.4861) centre (14.6867, 54.8115) ccw
  arc A283 (16.7222, 54.8056) -> (16.1766, 54.4861) centre (16.5967, 54.3944) ccw
  line L71 (16.7222, 54.8056) -> (17.7372, 54.4856)
  arc A284 (18.0009, 53.9109) -> (17.7372, 54.4856) centre (17.6041, 54.0767) ccw
  arc A285 (18.0009, 53.9109) -> (18.8864, 51.8898) centre (19.4079, 53.3229) ccw
  arc A286 (9.5889, 54.3811) -> (11.3662, 55.6887) centre (9.8537, 55.8829) ccw
  arc A287 (11.8819, 56.0545) -> (11.3662, 55.6887) centre (11.7927, 55.6339) ccw
  line L72 (11.8819, 56.0545) -> (12.921, 55.8242)
  arc A288 (13.2337, 55.2746) -> (12.921, 55.8242) centre (12.824, 55.4052) ccw
  arc A289 (13.2337, 55.2746) -> (14.292, 53.3384) centre (14.6867, 54.8115) ccw
  arc A290 (4.8127, 55.0099) -> (6.4694, 56.4674) centre (4.9457, 56.5291) ccw
  arc A291 (6.9512, 56.8768) -> (6.4694, 56.4674) centre (6.8991, 56.45) ccw
  line L73 (6.9512, 56.8768) -> (8.0064, 56.7379)
  arc A292 (8.3659, 56.2177) -> (8.0064, 56.7379) centre (7.9464, 56.3121) ccw
  arc A293 (8.3659, 56.2177) -> (9.5889, 54.3811) centre (9.8537, 55.8829) ccw
  line L74 (0, 0) -> (0, -55.22) construction
  line L75 (0, 0) -> (0.0096, -55.22) construction
  circle A294 centre (0, 0) radius 52.0383 construction
  arc A295 (0, -52.0483) -> (0.0091, -52.0482) centre (0, 0) ccw
  line L76 (0, -52.0483) -> (0, -52.0383)
  circle A296 centre (0, 0) radius 52.0383 projected
  line L77 (0.0091, -52.0482) -> (0.0091, -52.0382)
  point P0 (-54.3811, -9.5889)
  point P1 (-47.8219, -27.61)
  point P2 (-39.0464, -39.0464)
  point P3 (-35.4947, -42.301)
  point P4 (-27.61, -47.8219)
  point P5 (-18.8864, -51.8898)
  point P6 (-14.292, -53.3384)
  point P7 (-9.5889, -54.3811)
  point P8 (9.5889, -54.3811)
  point P9 (42.301, -35.4947)
  point P10 (50.0463, -23.337)
  point P11 (55.0099, 4.8127)
  point P12 (54.3811, 9.5889)
  point P13 (53.3384, 14.292)
  point P14 (47.8219, 27.61)
  point P15 (45.2336, 31.6729)
  point P16 (42.301, 35.4947)
  point P17 (39.0464, 39.0464)
  point P18 (35.4947, 42.301)
  point P19 (31.6729, 45.2336)
  point P20 (23.337, 50.0463)
  point P21 (14.292, 53.3384)
  point P22 (0, 55.22)
  point P23 (-31.6729, 45.2336)
  point P24 (-39.0464, 39.0464)
  point P25 (-45.2336, 31.6729)
  point P26 (-47.8219, 27.61)
  point P27 (-50.0463, 23.337)
  point P28 (-53.3384, 14.292)
  point P29 (-54.3811, 9.5889)
  dimension "d20" = 114.6
  dimension "d21" = 110.44
  dimension "d22" = 3.05
  dimension "d23" = 0.86
  dimension "d24" = 5
  dimension "d27" = 360
  dimension "d29" = 0.01
  dimension "d30" = 0.01
  constraints: 594 point on circle, 295 centre point, 156 end point, 8 point on line, 7 coincident, 6 tangent, 2 equal radius, 1 collinear, 1 vertical, 1081 other
  measures "d20" diameter of A0
  measures "d21" diameter of A1
  measures "d22" diameter of A2
  measures "d23" diameter of A3
  measures "d24" angle of L1 L0
  measures "d29" angle of L75 L74
  measures "d30" distance of L76.start L76.end
extrude "Extrusion2" add sketch "Sketch3" against normal up to surface (14 mm away)
sketch "Sketch4" plane through (0, 0, 14) normal (0, 0, 1) x (1, 0, 0)
  circle A0 centre (0, 0) radius 55.22
  arc A1 (-56.7329, 3.4343) -> (-56.4674, 6.4694) centre (-56.5291, 4.9457) ccw projected
  circle A2 centre (0, 0) radius 58.0975
  line L0 (-57.2198, 3.0309) -> (-57.2662, 1.9676) projected
  dimension "d44" = 0.8
  constraints: 2 centre point, 1 coincident, 1 tangent
  measures "d44" distance edge to line of A2 L0
extrude "Extrusion3" add sketch "Sketch4" against normal blind 1.5
sketch "Sketch6" plane through (0, 0, 0) normal (0, 1, 0) x (-1, 0, 0)
  circle A0 centre (51.435, 14.7937) radius 1.9844
  line L0 (58.0975, 14) -> (-58.0975, 14) projected
  line L1 (0, -4.3556) -> (0, 26.1338) projected
  point P0 (0, 0)
  point P1 (53.2537, 14)
  point P2 (49.6163, 14)
  dimension "d36" = 3.9688
  dimension "d37" = 0.7937
  dimension "d38" = 51.435
  constraints: 1 centre point
  measures "d36" diameter of A0
  measures "d37" distance from line of L0 A0.centre
  measures "d38" distance from line of L1 A0.centre
revolve "Revolution1" cut sketch "Sketch6" angle 360 about axis through (0, 0, 0) along (0, 0, 1) picked at (51.283, 13.6208) contours L0 A0
ref_plane "Work Plane4" through (0, 0, 7) normal (0, 0, 1) x (1, 0, 0)
chamfer "Chamfer1" distance 0.4 angle 45 1 edges at (-58.0975, 0, 12.5)
mirror "Mirror2" about plane through (0, 0, 7) normal (0, 0, 1) of "Revolution1", "Extrusion3", "Chamfer1"
equation "\"d0\" = 1.1 * da_df"
equation "\"d1\" = da_b"
equation "\"d3\" = da_dw"
equation "\"d15\" = da_aw"
equation "\"d19\" = da_aw"
equation "\"da_df\" = 94.615"
equation "\"da_b\" = 14"
equation "\"da_dw\" = 91.44"
equation "\"da_aw\" = 30.48"
body "Solid1"
body "Srf1"
